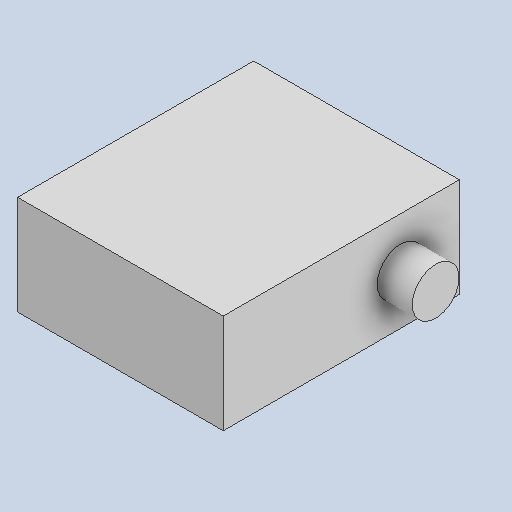
# Autodesk Inventor part: servo_cos
Saved by Autodesk Inventor 2022 (Build 260153000, 153)
## iProperties
Created: 2022-12-24
Part Number: servo_cos
Material: Generic
Document SubType Name: Modeling
Designer: Kamil
Density: 1 g/cm^3
Appearance: Default
Author: Kamil
Autodesk Inventor part; units mm, degrees
ref_plane "YZ Plane" through (0, 0, 0) normal (1, 0, 0) x (0, 1, 0)
ref_plane "XZ Plane" through (0, 0, 0) normal (0, 1, 0) x (-1, 0, 0)
ref_plane "XY Plane" through (0, 0, 0) normal (0, 0, 1) x (1, 0, 0)
sketch "Sketch1" plane through (0, 0, 0) normal (0, 1, 0) x (-1, 0, 0)
  line L0 (46.923, -68.9252) -> (29.323, -68.9252)
  line L1 (29.323, -68.9252) -> (29.323, -48.7252)
  line L2 (29.323, -48.7252) -> (46.923, -48.7252)
  line L3 (46.923, -48.7252) -> (46.923, -68.9252)
  point P0 (0, 0)
  dimension "d0" = 17.6
  dimension "d1" = 20.2
  constraints: 8 end point, 2 parallel, 1 horizontal, 1 perpendicular
  measures "d0" distance of L1.end L2.end
  measures "d1" distance of L0.end L1.end
extrude "Extrusion1" add sketch "Sketch1" along normal blind 8.5
sketch "Sketch2" plane through (-29.323, 0, -48.7252) normal (1, 0, 0) x (0, 0, -1)
  line L0 (0, 0) -> (20.2, 0) projected
  line L1 (20.2, 0) -> (20.2, 8.5) projected
  line L2 (0, 8.5) -> (20.2, 8.5) projected
  line L3 (0, 0) -> (0, 8.5) projected
  line L4 (20.2, 0) -> (20.2, 8.5) projected
  line L5 (20.2, 4.25) -> (0, 4.25)
  line L6 (0, 0) -> (0, 8.5) projected
  circle A0 centre (15.1699, 4.25) radius 2
  point P0 (-48.7252, 0)
  dimension "d4" = 4
  constraints: 2 end point, 2 midpoint, 1 centre point, 1 point on line
  measures "d4" diameter of A0
extrude "Extrusion2" add sketch "Sketch2" along normal blind 3 contours A0 L5 | L5 A0
body "Solid1"
